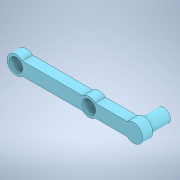
# Autodesk Inventor part: Component38
Saved by Autodesk Inventor 2022 (Build 260153000, 153)
## iProperties
Created: 2022-01-29
Part Number: Component38
Material: Generic
Document SubType Name: Modeling
Designer: Administrator
Density: 1 g/cm^3
Appearance: Default
Title: Component38
Author: Administrator
Autodesk Inventor part; units mm, degrees
ref_plane "YZ Plane" through (0, 0, 0) normal (1, 0, 0) x (0, 1, 0)
ref_plane "XZ Plane" through (0, 0, 0) normal (0, 1, 0) x (-1, 0, 0)
ref_plane "XY Plane" through (0, 0, 0) normal (0, 0, 1) x (1, 0, 0)
sketch "Sketch2" plane through (0, 0, 0) normal (0, 0, 1) x (1, 0, 0)
  circle A0 centre (-38.041, 5.7096) radius 3.25
  circle A1 centre (-2.041, 5.7096) radius 3.25
  circle A2 centre (19.959, 5.7096) radius 3.25
  arc A3 (16.8466, 2.4596) -> (16.8466, 8.9596) centre (19.959, 5.7096) ccw
  arc A4 (1.0715, 8.9596) -> (-5.1534, 8.9596) centre (-2.041, 5.7096) ccw
  line L0 (-5.1534, 8.9596) -> (-34.9285, 8.9596)
  arc A5 (-34.9285, 8.9596) -> (-34.9285, 2.4596) centre (-38.041, 5.7096) ccw
  arc A6 (-5.1534, 2.4596) -> (1.0715, 2.4596) centre (-2.041, 5.7096) ccw
  line L1 (1.0715, 8.9596) -> (16.8466, 8.9596)
  line L2 (-53.975, 5.7096) -> (31.1837, 5.7096) construction
  line L3 (-5.1534, 2.4596) -> (-34.9285, 2.4596)
  line L4 (1.0715, 2.4596) -> (16.8466, 2.4596)
  point P0 (0, 0)
  dimension "d4" = 22
  dimension "d5" = 36
  dimension "d6" = 6.5
  dimension "d7" = 9
  dimension "d8" = 6.5
  constraints: 10 end point, 8 point on circle, 7 centre point, 5 equal radius, 4 coincident, 4 horizontal, 4 symmetric about line, 3 point on line, 1 collinear
  measures "d4" distance of A2.centre A1.centre
  measures "d5" distance of A1.centre A0.centre
  measures "d6" diameter of A0
  measures "d7" diameter of A5
  measures "d8" distance between parallel lines of L3 L0
extrude "Extrusion1" add sketch "Sketch2" along normal blind 5 contours A2 | L4 A6 L3 A5 L0 A4 L1 A3
extrude "Extrusion2" add sketch "Sketch2" against normal blind 10 contours A2
equation "\"d6\" = R"
equation "\"d7\" = R1"
equation "\"d8\" = width"
equation "\"d0\" = thickness"
equation "\"d2\" = 2 * thickness"
equation "\"R\" = 6.5"
equation "\"thickness\" = 5"
equation "\"width\" = 6.5"
equation "\"R1\" = 9"
body "Solid1"
